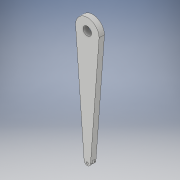
# Autodesk Inventor part: Jambe
Saved by Autodesk Inventor 2019 (Build 230136000, 136)
## iProperties
Created: 2020-01-16
Part Number: Jambe
Material: Générique
Document SubType Name: Modeling
Designer: Quentin
Density: 1 g/cm^3
Appearance: Par défaut
Author: Quentin
Autodesk Inventor part; units mm, degrees
ref_plane "YZ Plane" through (0, 0, 0) normal (1, 0, 0) x (0, 1, 0)
ref_plane "XZ Plane" through (0, 0, 0) normal (0, 1, 0) x (-1, 0, 0)
ref_plane "XY Plane" through (0, 0, 0) normal (0, 0, 1) x (1, 0, 0)
sketch "Esquisse1" plane through (0, 0, 0) normal (0, 0, 1) x (1, 0, 0)
  arc A0 (22.8757, 107.3508) -> (1.1243, 107.3508) centre (12, 109) ccw
  arc A1 (9.0085, 2.7745) -> (14.9915, 2.7745) centre (12, 3) ccw
  line L0 (1, 109) -> (9.0085, 2.7745)
  line L1 (23, 109) -> (14.9915, 2.7745)
  point P0 (0, 0)
  dimension "d2" = 22
  constraints: 6 point on circle, 4 end point, 2 centre point, 2 point on line, 2 tangent
  measures "d2" diameter of A0
extrude "Extrusion1" add sketch "Esquisse1" along normal blind 5 contours L1 A1 L0 A0
sketch "Esquisse2" plane through (23, 109, 5) normal (0.9971701, -0.075178, 0) x (0, 0, -1)
  line L0 (5, -109.527) -> (0, -109.527) projected
  line L1 (2.5, -109.527) -> (1.5, -109.527)
  line L2 (2.5, -109.527) -> (3.5, -109.527)
  line L3 (3.5, -109.527) -> (3.5, -104.527)
  line L4 (3.5, -104.527) -> (1.5, -104.527)
  line L5 (1.5, -104.527) -> (1.5, -109.527)
  point P0 (5, -110.4206)
  dimension "d6" = 1
  dimension "d7" = 1
  dimension "d8" = 5
  dimension "d9" = 2
  constraints: 10 end point, 2 perpendicular, 2 point on line, 1 midpoint
  measures "d6" distance of L1.start L1.end
  measures "d7" distance of L1.start L2.end
  measures "d8" distance of L2.end L3.end
  measures "d9" distance of L3.end L4.end
extrude "Extrusion2" cut sketch "Esquisse2" against normal through all
sketch "Esquisse3" plane through (0, 0, 0) normal (0, 0, -1) x (-1, 0, 0)
  arc A0 (-14.9915, 2.7745) -> (-9.0085, 2.7745) centre (-12, 3) ccw projected
  arc A1 (-1, 109) -> (-23, 109) centre (-12, 109) ccw projected
  circle A2 centre (-12, 109) radius 4
  arc A3 (-14.9915, 2.7745) -> (-9.0085, 2.7745) centre (-12, 3) ccw projected
  line L0 (-12, 0) -> (-12, 2)
  circle A4 centre (-12, 2) radius 1
  line L1 (-14.8284, 2) -> (-9.1716, 2)
  point P0 (0, 0)
  dimension "d13" = 8
  dimension "d24" = 2
  dimension "d25" = 2
  dimension "d26" = 5.6569
  constraints: 4 end point, 4 point on circle, 2 centre point, 2 coincident, 1 horizontal, 1 vertical
  measures "d13" diameter of A2
  measures "d24" distance of L0.start L0.end
  measures "d25" diameter of A4
  measures "d26" distance of L1.start L1.end
extrude "Extrusion3" cut sketch "Esquisse3" against normal through all contours L1 L0 A4 | A4 L1 | L0 L1 A4 | A2
